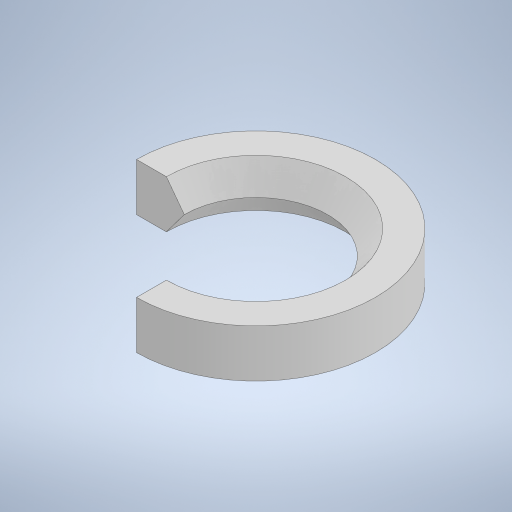
# Autodesk Inventor part: C-ClipV1
Saved by Autodesk Inventor 2024 (Build 280153000, 153)
## iProperties
Created: 2024-01-02
Part Number: C-ClipV1
Material: Generisch
Document SubType Name: Modeling
Designer: chris
Density: 1 g/cm^3
Appearance: Vorgabe
Author: chris
Autodesk Inventor part; units mm, degrees
ref_plane "YZ Plane" through (0, 0, 0) normal (1, 0, 0) x (0, 1, 0)
ref_plane "XZ Plane" through (0, 0, 0) normal (0, 1, 0) x (-1, 0, 0)
ref_plane "XY Plane" through (0, 0, 0) normal (0, 0, 1) x (1, 0, 0)
sketch "Skizze1" plane through (0, 0, 0) normal (0, 0, 1) x (1, 0, 0)
  circle A0 centre (0, 0) radius 7.5
  circle A1 centre (0, 0) radius 10
  line L0 (0, 0) -> (-10, 0)
  line L1 (0, 0) -> (0, -10)
  point P0 (0, -7.5)
  point P1 (-7.5, 0)
  dimension "d0" = 15
  dimension "d1" = 20
  constraints: 4 end point, 2 centre point, 2 coincident, 2 point on circle, 1 horizontal, 1 perpendicular
  measures "d0" diameter of A0
  measures "d1" diameter of A1
extrude "Extrusion1" add sketch "Skizze1" along normal blind 4 contours A0 L0 A1 L1 picked at (-8.9972, 1.396)
sketch "Skizze2" plane through (-10, 0, 0) normal (0, -1, 0) x (1, 0, 0)
  line L0 (2.5, 0) -> (2.5, 4) construction
  line L1 (2.5, 2) -> (4, 2) construction
  line L2 (4, 2) -> (2.5, 4)
  line L3 (20, 4) -> (0, 4) projected
  line L4 (4, 2) -> (2.5, 0)
  line L5 (2.5, 0) -> (2.5, 4)
  line L6 (10, -0.8) -> (10, 4.8) projected
  point P0 (10, 0)
  point P1 (10, 4)
  dimension "d4" = 1.5
  constraints: 8 end point, 1 horizontal, 1 midpoint, 1 perpendicular, 1 point on line
  measures "d4" distance of L1.start L1.end
revolve "Umdrehung1" add sketch "Skizze2" angle 270 about axis through (0, 0, -10) along (0, 0, -1)
